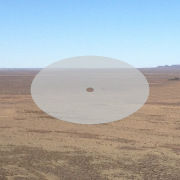
# Autodesk Inventor part: 2f3surf
Saved by Autodesk Inventor 2013 SP2 (Build 170200200, 200)
## iProperties
Company: HERA Project
Created: 2013-05-29
Part Number: 2f3surf
Material: Glass
Document SubType Name: Modeling
Designer: David DeBoer
Density: 2.18 g/cm^3
Description: Feed backplane conducting surface
Mass: 8147.17 g
Surface Area: 29543.6 cm^2
Volume: 3737.23 cm^3
Author: David DeBoer
Title: Feed backplane surface
Autodesk Inventor part; units mm, degrees
ref_plane "YZ Plane" through (0, 0, 0) normal (1, 0, 0) x (0, 1, 0)
ref_plane "XZ Plane" through (0, 0, 0) normal (0, 1, 0) x (-1, 0, 0)
ref_plane "XY Plane" through (0, 0, 0) normal (0, 0, 1) x (1, 0, 0)
sketch "Sketch1" plane through (0, 0, 0) normal (0, 1, 0) x (-1, 0, 0)
  circle A0 centre (0.5489, 0.4288) radius 685.8
  point P0 (0, 0)
  dimension "d0" = 1371.6
  constraints: 1 centre point
  measures "d0" diameter of A0
extrude "Extrusion1" add sketch "Sketch1" along normal blind 2.54
sketch "Sketch2" plane through (-0.5489, 2.54, 0.4288) normal (0, 1, 0) x (1, 0, 0)
  circle A0 centre (0.5489, 0.4288) radius 44.45
  dimension "d7" = 88.9
  constraints: 1 centre point, 1 coincident
  measures "d7" diameter of A0
extrude "Extrusion2" cut sketch "Sketch2" against normal blind 25.4
body "Solid1"
